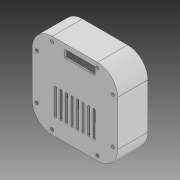
# Autodesk Inventor part: J1_Base
Saved by Autodesk Inventor 2020 (Build 240168000, 168)
## iProperties
Created: 2021-03-23
Part Number: J1_Base
Material: Generic
Document SubType Name: Modeling
Designer: DDeGo
Density: 1 g/cm^3
Appearance: Default
Author: DDeGo
Autodesk Inventor part; units mm, degrees
ref_plane "YZ Plane" through (0, 0, 0) normal (1, 0, 0) x (0, 1, 0)
ref_plane "XZ Plane" through (0, 0, 0) normal (0, 1, 0) x (-1, 0, 0)
ref_plane "XY Plane" through (0, 0, 0) normal (0, 0, 1) x (1, 0, 0)
sketch "Block1" plane through (0, 0, 0) normal (0, 0, 1) x (1, 0, 0)
  circle A0 centre (112.1187, 97.7562) radius 2.75
  line L0 (90.8687, 90.2562) -> (90.8687, 49.9679) construction
  circle A1 centre (83.3687, 50.2562) radius 2.75
  line L1 (75.8687, 49.9679) -> (75.8687, 122.7562) construction
  line L2 (75.8687, 49.9679) -> (90.8687, 49.9679) construction
  circle A2 centre (83.3687, 115.2562) radius 2.75
  line L3 (90.8687, 90.2562) -> (190.8687, 90.2562) construction
  line L4 (75.8687, 122.7562) -> (205.8687, 122.7562) construction
  circle A3 centre (140.8687, 115.2562) radius 2.75
  circle A4 centre (169.6187, 97.7562) radius 2.75
  circle A5 centre (198.3687, 115.2562) radius 2.75
  line L5 (190.8687, 90.2562) -> (190.8687, 40.2562) construction
  line L6 (205.8687, 40.2562) -> (205.8687, 122.7562) construction
  circle A6 centre (198.3687, 50.2562) radius 2.75
  line L7 (205.8687, 40.2562) -> (190.8687, 40.2562) construction
  line L8 (83.3687, 115.2562) -> (140.8687, 115.2562) construction
  line L9 (140.8687, 115.2562) -> (198.3687, 115.2562) construction
  line L10 (198.3687, 115.2562) -> (198.3687, 50.2562) construction
  line L11 (198.3687, 50.2562) -> (83.3687, 50.2562) construction
  line L12 (83.3687, 50.2562) -> (83.3687, 115.2562) construction
  line L13 (112.1187, 115.2562) -> (112.1187, 97.7562) construction
  line L14 (169.6187, 115.2562) -> (169.6187, 97.7562) construction
  line L15 (169.6187, 97.7562) -> (112.1187, 97.7562) construction
  point P0 (142.3997, 87.8737)
  point P1 (140.8687, 90.2562)
  point P2 (140.8687, 90.2562)
  dimension "d9" = 5.5
  dimension "d10" = 57.5
  dimension "d11" = 7.5
  dimension "d12" = 7.5
  dimension "d13" = 7.5
  dimension "d14" = 17.5
  dimension "d15" = 7.5
  dimension "d16" = 10
  dimension "d17" = 65
  dimension "d18" = 7.5
  dimension "d19" = 7.5
  measures "d9" diameter of A0
  measures "d10" distance of L8.start L8.end
  measures "d11" distance between parallel lines of L6 L10
  measures "d12" distance between parallel lines of L4 L9
  measures "d13" distance between parallel lines of L1 L12
  measures "d14" distance of L13.start L13.end
  measures "d15" distance between parallel lines of L3 L15
  measures "d16" distance between parallel lines of L7 L11
  measures "d17" distance of L9.end L10.end
  measures "d18" distance from line of L5 L10.end
  measures "d19" distance between parallel lines of L12 L0
sketch "Sketch1" plane through (0, 0, 0) normal (0, 0, 1) x (1, 0, 0)
  line L0 (45, -85) -> (-45, -85)
  line L1 (-85, -45) -> (-85, 45)
  line L2 (-45, 85) -> (45, 85)
  line L3 (85, 45) -> (85, -45)
  line L4 (85, -85) -> (-85, 85) construction
  line L5 (-85, -85) -> (85, 85) construction
  arc A0 (-45, 85) -> (-85, 45) centre (-45, 45) ccw
  arc A1 (85, 45) -> (45, 85) centre (45, 45) ccw
  arc A2 (45, -85) -> (85, -45) centre (45, -45) ccw
  arc A3 (-85, -45) -> (-45, -85) centre (-45, -45) ccw
  point P0 (0, 0)
  dimension "d1" = 170
  dimension "d2" = 170
  dimension "d3" = 40
  constraints: 12 end point, 8 point on circle, 8 point on line, 8 tangent, 4 centre point, 3 equal radius, 2 midpoint, 2 parallel, 1 horizontal, 1 perpendicular
  measures "d1" distance between parallel lines of L3 L1
  measures "d2" distance between parallel lines of L0 L2
  measures "d3" radius of A0
extrude "Extrusion1" add sketch "Sketch1" along normal blind 60
sketch "Sketch2" plane through (0, 0, 60) normal (0, 0, 1) x (1, 0, 0)
  line L0 (0, 0) -> (-85, 0) construction
  line L1 (-85, 45) -> (-85, -45) projected
  line L2 (0, 0) -> (0, 52.5) construction
  line L3 (45, 85) -> (-45, 85) projected
  circle A0 centre (-28.75, 60) radius 2.75
  line L4 (-50, 52.5) -> (-50, 12.2116) construction
  circle A1 centre (-57.5, 12.5) radius 2.75
  line L5 (-65, 12.2116) -> (-65, 85) construction
  line L6 (-65, 12.2116) -> (-50, 12.2116) construction
  circle A2 centre (-57.5, 77.5) radius 2.75
  line L7 (-50, 52.5) -> (50, 52.5) construction
  line L8 (-65, 85) -> (65, 85) construction
  circle A3 centre (0, 77.5) radius 2.75
  circle A4 centre (28.75, 60) radius 2.75
  circle A5 centre (57.5, 77.5) radius 2.75
  line L9 (50, 52.5) -> (50, 2.5) construction
  line L10 (65, 2.5) -> (65, 85) construction
  circle A6 centre (57.5, 12.5) radius 2.75
  line L11 (65, 2.5) -> (50, 2.5) construction
  line L12 (-57.5, 77.5) -> (0, 77.5) construction
  line L13 (0, 77.5) -> (57.5, 77.5) construction
  line L14 (57.5, 77.5) -> (57.5, 12.5) construction
  line L15 (57.5, 12.5) -> (-57.5, 12.5) construction
  line L16 (-57.5, 12.5) -> (-57.5, 77.5) construction
  line L17 (-28.75, 77.5) -> (-28.75, 60) construction
  line L18 (28.75, 77.5) -> (28.75, 60) construction
  line L19 (28.75, 60) -> (-28.75, 60) construction
  circle A7 centre (-28.75, -60) radius 2.75
  line L20 (-50, -52.5) -> (-50, -12.2116) construction
  circle A8 centre (-57.5, -12.5) radius 2.75
  line L21 (-65, -12.2116) -> (-65, -85) construction
  line L22 (-65, -12.2116) -> (-50, -12.2116) construction
  circle A9 centre (-57.5, -77.5) radius 2.75
  line L23 (-50, -52.5) -> (50, -52.5) construction
  line L24 (-65, -85) -> (65, -85) construction
  circle A10 centre (0, -77.5) radius 2.75
  circle A11 centre (28.75, -60) radius 2.75
  circle A12 centre (57.5, -77.5) radius 2.75
  line L25 (50, -52.5) -> (50, -2.5) construction
  line L26 (65, -2.5) -> (65, -85) construction
  circle A13 centre (57.5, -12.5) radius 2.75
  line L27 (65, -2.5) -> (50, -2.5) construction
  line L28 (-57.5, -77.5) -> (0, -77.5) construction
  line L29 (0, -77.5) -> (57.5, -77.5) construction
  line L30 (57.5, -77.5) -> (57.5, -12.5) construction
  line L31 (57.5, -12.5) -> (-57.5, -12.5) construction
  line L32 (-57.5, -12.5) -> (-57.5, -77.5) construction
  line L33 (-28.75, -77.5) -> (-28.75, -60) construction
  line L34 (28.75, -77.5) -> (28.75, -60) construction
  line L35 (28.75, -60) -> (-28.75, -60) construction
  constraints: 4 end point, 2 horizontal, 1 midpoint, 1 vertical, 2 other
extrude "Extrusion2" [suppressed]
ref_plane "Work Plane1" through (0, 0, -15) normal (0, 0, -1) x (-1, 0, 0)
sketch "Sketch3" plane through (0, 0, -15) normal (0, 0, -1) x (-1, 0, 0)
  circle A0 centre (0, 0) radius 87.5
  line L0 (-85, -45) -> (-85, 45) construction
  dimension "d27" = 175
  constraints: 1 centre point, 1 coincident
  measures "d27" diameter of A0
sketch "Sketch4" plane through (0, 0, 0) normal (0, 0, -1) x (-1, 0, 0)
  line L0 (-85, -45) -> (-85, 45) projected
  arc A0 (-85, -45) -> (-45, -85) centre (-45, -45) ccw projected
  line L1 (45, -85) -> (-45, -85) projected
  arc A1 (45, -85) -> (85, -45) centre (45, -45) ccw projected
  line L2 (85, 45) -> (85, -45) projected
  arc A2 (85, 45) -> (45, 85) centre (45, 45) ccw projected
  line L3 (-45, 85) -> (45, 85) projected
  arc A3 (-45, 85) -> (-85, 45) centre (-45, 45) ccw projected
  point P0 (0, 0)
loft "Loft1" add profiles "Sketch3", "Sketch4"
sketch "Sketch5" plane through (0, 0, -15) normal (0, 0, -1) x (-1, 0, 0)
  arc A0 (-37.1204, 79.2359) -> (-77.3314, 40.9402) centre (0, 0) ccw projected
  arc A1 (-77.3314, 40.9402) -> (-77.3314, -40.9402) centre (0, 0) ccw projected
  arc A2 (-77.3314, -40.9402) -> (-40.9402, -77.3314) centre (0, 0) ccw projected
  arc A3 (-40.9402, -77.3314) -> (40.9402, -77.3314) centre (0, 0) ccw projected
  arc A4 (40.9402, -77.3314) -> (77.3314, -40.9402) centre (0, 0) ccw projected
  arc A5 (77.3314, -40.9402) -> (77.3314, 40.9402) centre (0, 0) ccw projected
  arc A6 (77.3314, 40.9402) -> (40.9402, 77.3314) centre (0, 0) ccw projected
  arc A7 (40.9402, 77.3314) -> (-37.1204, 79.2359) centre (0, 0) ccw projected
extrude "Extrusion3" add sketch "Sketch5" along normal blind 5
ref_plane "Work Plane2" through (0, 0, 57) normal (0, 0, 1) x (1, 0, 0)
sketch "Sketch6" plane through (0, 0, 57) normal (0, 0, 1) x (1, 0, 0)
  arc A0 (-45, 85) -> (-85, 45) centre (-45, 45) ccw projected
  line L0 (-85, 45) -> (-85, -45) projected
  arc A1 (-85, -45) -> (-45, -85) centre (-45, -45) ccw projected
  line L1 (-45, -85) -> (45, -85) projected
  arc A2 (45, -85) -> (85, -45) centre (45, -45) ccw projected
  line L2 (85, -45) -> (85, 45) projected
  arc A3 (85, 45) -> (45, 85) centre (45, 45) ccw projected
  line L3 (45, 85) -> (-45, 85) projected
  line L4 (-81, -45) -> (-81, 45)
  arc A4 (-45, 81) -> (-81, 45) centre (-45, 45) ccw
  line L5 (-45, 81) -> (45, 81)
  arc A5 (81, 45) -> (45, 81) centre (45, 45) ccw
  line L6 (81, 45) -> (81, -45)
  arc A6 (45, -81) -> (81, -45) centre (45, -45) ccw
  line L7 (45, -81) -> (-45, -81)
  arc A7 (-81, -45) -> (-45, -81) centre (-45, -45) ccw
  line L8 (-85, 45) -> (-85, -45) projected
  point P0 (0, 0)
  dimension "d29" = 4
  constraints: 8 end point, 8 point on circle, 4 centre point, 7 other
  measures "d29" distance between parallel lines of L8 L4
ref_plane "Work Plane3" through (85, -45, 0) normal (0, 0, -1) x (-1, 0, 0)
sketch "Sketch7" plane through (85, -45, 0) normal (0, 0, -1) x (-1, 0, 0)
  arc A0 (170, 90) -> (130, 130) centre (130, 90) ccw projected
  line L0 (170, 90) -> (170, 0) projected
  arc A1 (130, -40) -> (170, 0) centre (130, 0) ccw projected
  line L1 (130, -40) -> (40, -40) projected
  arc A2 (0, 0) -> (40, -40) centre (40, 0) ccw projected
  line L2 (0, 0) -> (0, 90) projected
  arc A3 (40, 130) -> (0, 90) centre (40, 90) ccw projected
  line L3 (40, 130) -> (130, 130) projected
  line L4 (166, 0) -> (166, 90)
  arc A4 (166, 90) -> (130, 126) centre (130, 90) ccw
  line L5 (130, 126) -> (40, 126)
  arc A5 (40, 126) -> (4, 90) centre (40, 90) ccw
  line L6 (4, 90) -> (4, 0)
  arc A6 (4, 0) -> (40, -36) centre (40, 0) ccw
  line L7 (40, -36) -> (130, -36)
  arc A7 (130, -36) -> (166, 0) centre (130, 0) ccw
  point P0 (85, 45)
  dimension "d30" = 4
  constraints: 8 end point, 8 point on circle, 4 centre point, 7 other
  measures "d30" distance between parallel lines of L0 L4
extrude "Extrusion4" cut sketch "Sketch6" against normal up to surface (57 mm away) contours L4 A4 L5 A5 L6 A6 L7 A7
sketch "Sketch8" plane through (0, 0, -20) normal (0, 0, -1) x (-1, 0, 0)
  circle A0 centre (0, 0) radius 72.5
  dimension "d33" = 145
  constraints: 1 centre point, 1 coincident
  measures "d33" diameter of A0
extrude "Extrusion5" cut sketch "Sketch8" against normal blind 29.75
sketch "Sketch9" plane through (-81, -45, 57) normal (-1, 0, 0) x (0, 0, 1)
  line L0 (-13.6892, 69.9987) -> (-53.6892, 69.9987) construction
  line L1 (-53.6892, 69.9987) -> (-53.6892, 29.9987) construction
  line L2 (-53.6892, 29.9987) -> (-13.6892, 29.9987) construction
  line L3 (-13.6892, 29.9987) -> (-13.6892, 69.9987) construction
  line L4 (-13.6892, 69.9987) -> (-53.6892, 29.9987) construction
  line L5 (-53.6892, 69.9987) -> (-13.6892, 29.9987) construction
  circle A0 centre (-33.6892, 49.9987) radius 19
  point P0 (-57, 45)
  dimension "d36" = 40
  dimension "d37" = 40
  dimension "d38" = 38
  constraints: 12 end point, 2 midpoint, 2 parallel, 1 centre point, 1 coincident, 1 horizontal, 1 perpendicular
  measures "d36" distance of L0.end L1.end
  measures "d37" distance of L1.end L2.end
  measures "d38" diameter of A0
extrude "Extrusion6" cut sketch "Sketch9" along normal through all
sketch "Sketch10" plane through (0, 0, 57) normal (0, 0, -1) x (-1, 0, 0)
  line L0 (20, 60.5) -> (-40, 60.5)
  line L1 (-40, 60.5) -> (-40, 75.4)
  line L2 (-40, 75.4) -> (20, 75.4)
  line L3 (20, 75.4) -> (20, 60.5)
  line L4 (-45, 85) -> (45, 85) projected
  point P0 (0, 0)
  point P1 (0, 85)
  dimension "d69" = 9.6
  dimension "d70" = 24.5
  dimension "d71" = 20
  dimension "d72" = 40
  constraints: 8 end point, 2 parallel, 1 horizontal, 1 midpoint, 1 perpendicular
  measures "d69" distance between parallel lines of L4 L2
  measures "d70" distance between parallel lines of L4 L0
  measures "d71" distance from line of L3 point (0, 85)
  measures "d72" distance from line of L1 point (0, 85)
extrude "Extrusion7" cut sketch "Sketch10" against normal through all
sketch "Sketch11" plane through (0, 0, 60) normal (0, 0, 1) x (1, 0, 0)
  line L0 (-38.2933, -49.6427) -> (-38.2933, 0.3573) construction
  line L1 (-40.2933, -49.6427) -> (-40.2933, 0.3573)
  line L2 (-36.2933, 0.3573) -> (-36.2933, -49.6427)
  arc A0 (-40.2933, -49.6427) -> (-36.2933, -49.6427) centre (-38.2933, -49.6427) ccw
  arc A1 (-36.2933, 0.3573) -> (-40.2933, 0.3573) centre (-38.2933, 0.3573) ccw
  line L3 (0, 0) -> (68.8945, 0) construction
  line L4 (-27.2933, -49.6427) -> (-27.2933, 0.3573) construction
  line L5 (-29.2933, -49.6427) -> (-29.2933, 0.3573)
  line L6 (-25.2933, 0.3573) -> (-25.2933, -49.6427)
  arc A2 (-29.2933, -49.6427) -> (-25.2933, -49.6427) centre (-27.2933, -49.6427) ccw
  arc A3 (-25.2933, 0.3573) -> (-29.2933, 0.3573) centre (-27.2933, 0.3573) ccw
  line L7 (-16.2933, -49.6427) -> (-16.2933, 0.3573) construction
  line L8 (-18.2933, -49.6427) -> (-18.2933, 0.3573)
  line L9 (-14.2933, 0.3573) -> (-14.2933, -49.6427)
  arc A4 (-18.2933, -49.6427) -> (-14.2933, -49.6427) centre (-16.2933, -49.6427) ccw
  arc A5 (-14.2933, 0.3573) -> (-18.2933, 0.3573) centre (-16.2933, 0.3573) ccw
  line L10 (-5.2933, -49.6427) -> (-5.2933, 0.3573) construction
  line L11 (-7.2933, -49.6427) -> (-7.2933, 0.3573)
  line L12 (-3.2933, 0.3573) -> (-3.2933, -49.6427)
  arc A6 (-7.2933, -49.6427) -> (-3.2933, -49.6427) centre (-5.2933, -49.6427) ccw
  arc A7 (-3.2933, 0.3573) -> (-7.2933, 0.3573) centre (-5.2933, 0.3573) ccw
  line L13 (5.7067, -49.6427) -> (5.7067, 0.3573) construction
  line L14 (3.7067, -49.6427) -> (3.7067, 0.3573)
  line L15 (7.7067, 0.3573) -> (7.7067, -49.6427)
  arc A8 (3.7067, -49.6427) -> (7.7067, -49.6427) centre (5.7067, -49.6427) ccw
  arc A9 (7.7067, 0.3573) -> (3.7067, 0.3573) centre (5.7067, 0.3573) ccw
  line L16 (16.7067, -49.6427) -> (16.7067, 0.3573) construction
  line L17 (14.7067, -49.6427) -> (14.7067, 0.3573)
  line L18 (18.7067, 0.3573) -> (18.7067, -49.6427)
  arc A10 (14.7067, -49.6427) -> (18.7067, -49.6427) centre (16.7067, -49.6427) ccw
  arc A11 (18.7067, 0.3573) -> (14.7067, 0.3573) centre (16.7067, 0.3573) ccw
  line L19 (27.7067, -49.6427) -> (27.7067, 0.3573) construction
  line L20 (25.7067, -49.6427) -> (25.7067, 0.3573)
  line L21 (29.7067, 0.3573) -> (29.7067, -49.6427)
  arc A12 (25.7067, -49.6427) -> (29.7067, -49.6427) centre (27.7067, -49.6427) ccw
  arc A13 (29.7067, 0.3573) -> (25.7067, 0.3573) centre (27.7067, 0.3573) ccw
  line L22 (38.7067, -49.6427) -> (38.7067, 0.3573) construction
  line L23 (36.7067, -49.6427) -> (36.7067, 0.3573)
  line L24 (40.7067, 0.3573) -> (40.7067, -49.6427)
  arc A14 (36.7067, -49.6427) -> (40.7067, -49.6427) centre (38.7067, -49.6427) ccw
  arc A15 (40.7067, 0.3573) -> (36.7067, 0.3573) centre (38.7067, 0.3573) ccw
  point P0 (-38.2933, -24.6427)
  point P1 (-27.2933, -24.6427)
  point P2 (-16.2933, -24.6427)
  point P3 (-5.2933, -24.6427)
  point P4 (5.7067, -24.6427)
  point P5 (16.7067, -24.6427)
  point P6 (27.7067, -24.6427)
  point P7 (38.7067, -24.6427)
  dimension "d43" = 50
  dimension "d44" = 2
  dimension "d47" = 11
  constraints: 66 end point, 32 point on circle, 16 centre point, 4 tangent, 2 horizontal, 1 midpoint, 1 parallel, 1 vertical, 84 other
  measures "d43" distance of L0.start L0.end
  measures "d44" radius of A1
  measures "d47" distance of L1.start L5.start
extrude "Extrusion8" cut sketch "Sketch11" against normal blind 10
sketch "Sketch12" plane through (-45, 81, 0) normal (0, 0, 1) x (1, 0, 0)
  circle A0 centre (38.7385, -72.8833) radius 193.3593
  point P0 (45, -81)
  constraints: 1 centre point
extrude "SnipSnip" cut sketch "Sketch12" against normal through all
sketch "Sketch13" plane through (-45, -85, 60) normal (0, -1, 0) x (1, 0, 0)
  line L0 (-0.9101, -8.6737) -> (19.7466, -8.6737)
  line L1 (19.7466, -8.6737) -> (19.7466, -23.4777)
  line L2 (19.7466, -23.4777) -> (-0.9101, -23.4777)
  line L3 (-0.9101, -23.4777) -> (-0.9101, -8.6737)
  line L4 (61.8635, -8.6737) -> (77.0118, -8.6737)
  line L5 (77.0118, -8.6737) -> (77.0118, -15.7888)
  line L6 (77.0118, -15.7888) -> (61.8635, -15.7888)
  line L7 (61.8635, -15.7888) -> (61.8635, -8.6737)
  point P0 (45, -60)
  constraints: 16 end point, 4 parallel, 2 horizontal, 2 perpendicular, 1 point on line
extrude "Extrusion10" cut sketch "Sketch13" against normal blind 10
sketch "Sketch14" plane through (-45, 81, 0) normal (0, 0, -1) x (-1, 0, 0)
  arc A0 (0, -162) -> (36, -126) centre (0, -126) ccw projected
  line L0 (0, -162) -> (-90, -162) projected
  arc A1 (-126, -126) -> (-90, -162) centre (-90, -126) ccw projected
  line L1 (-126, -126) -> (-126, -36) projected
  arc A2 (-90, 0) -> (-126, -36) centre (-90, -36) ccw projected
  line L2 (-90, 0) -> (0, 0) projected
  arc A3 (36, -36) -> (0, 0) centre (0, -36) ccw projected
  line L3 (36, -36) -> (36, -126) projected
  arc A4 (-90, 4) -> (-130, -36) centre (-90, -36) ccw projected
  line L4 (-130, -126) -> (-130, -36) projected
  arc A5 (-130, -126) -> (-90, -166) centre (-90, -126) ccw projected
  line L5 (0, -166) -> (-90, -166) projected
  arc A6 (0, -166) -> (40, -126) centre (0, -126) ccw projected
  line L6 (40, -36) -> (40, -126) projected
  arc A7 (40, -36) -> (0, 4) centre (0, -36) ccw projected
  line L7 (-90, 4) -> (0, 4) projected
  line L8 (-90, -36) -> (-90, -5.5) construction
  line L9 (-90, -36) -> (-120.5, -36) construction
  line L10 (-90, -36) -> (-45, -81) construction
  circle A8 centre (-120.5, -36) radius 3.1
  circle A9 centre (-90, -5.5) radius 3.1
  arc A10 (-95.5, -5.5) -> (-84.5, -5.5) centre (-90, -5.5) ccw
  line L11 (-90, 0) -> (0, 0) projected
  arc A11 (-120.5, -41.5) -> (-120.5, -30.5) centre (-120.5, -36) ccw
  line L12 (-126, -126) -> (-126, -36) projected
  line L13 (-120.5, -41.5) -> (-126, -41.5)
  line L14 (-120.5, -30.5) -> (-126, -30.5)
  line L15 (-95.5, -5.5) -> (-95.5, 0)
  line L16 (-84.5, -5.5) -> (-84.5, 0)
  line L17 (-84.5, -156.5) -> (-84.5, -162)
  arc A12 (-84.5, -156.5) -> (-95.5, -156.5) centre (-90, -156.5) ccw
  line L18 (-95.5, -156.5) -> (-95.5, -162)
  circle A13 centre (-90, -156.5) radius 3.1
  line L19 (-120.5, -120.5) -> (-126, -120.5)
  arc A14 (-120.5, -131.5) -> (-120.5, -120.5) centre (-120.5, -126) ccw
  circle A15 centre (-120.5, -126) radius 3.1
  line L20 (-120.5, -131.5) -> (-126, -131.5)
  line L21 (30.5, -120.5) -> (36, -120.5)
  arc A16 (30.5, -120.5) -> (30.5, -131.5) centre (30.5, -126) ccw
  line L22 (30.5, -131.5) -> (36, -131.5)
  circle A17 centre (30.5, -126) radius 3.1
  line L23 (-5.5, -156.5) -> (-5.5, -162)
  arc A18 (5.5, -156.5) -> (-5.5, -156.5) centre (0, -156.5) ccw
  circle A19 centre (0, -156.5) radius 3.1
  line L24 (5.5, -156.5) -> (5.5, -162)
  line L25 (-5.5, -5.5) -> (-5.5, 0)
  arc A20 (-5.5, -5.5) -> (5.5, -5.5) centre (0, -5.5) ccw
  line L26 (5.5, -5.5) -> (5.5, 0)
  circle A21 centre (0, -5.5) radius 3.1
  line L27 (30.5, -41.5) -> (36, -41.5)
  arc A22 (30.5, -30.5) -> (30.5, -41.5) centre (30.5, -36) ccw
  circle A23 centre (30.5, -36) radius 3.1
  line L28 (30.5, -30.5) -> (36, -30.5)
  point P0 (-90, -162)
  point P1 (-90, -166)
  point P2 (-126, -126)
  point P3 (-130, -126)
  point P4 (36, -126)
  point P5 (40, -126)
  point P6 (0, -166)
  point P7 (0, 0)
  point P8 (0, 4)
  point P9 (36, -36)
  point P10 (40, -36)
  point P11 (36, -41.5)
  point P12 (35.5774, -30.5)
  point P13 (35.5774, -131.5)
  point P14 (36, -120.5)
  point P15 (-125.5774, -131.5)
  point P16 (-125.5774, -30.5)
  point P17 (-126, -41.5)
  point P18 (-84.5, 0)
  point P19 (-95.5, -0.4226)
  point P20 (5.5, -0.4226)
  point P21 (-5.5, 0)
  point P22 (-5.5, -162)
  point P23 (5.5, -161.5774)
  point P24 (-95.5, -161.5774)
  point P25 (-84.5, -162)
  dimension "d58" = 5.5
  dimension "d59" = 45
  dimension "d60" = 6.2
  dimension "d63" = 360
  dimension "d73" = 9.5
  constraints: 38 end point, 16 centre point, 16 coincident, 16 point on circle, 6 tangent, 5 perpendicular, 4 point on line, 1 equal radius, 106 other
  measures "d58" distance from line of L2 L8.end
  measures "d59" angle of L10 L8
  measures "d60" diameter of A9
  measures "d73" distance from line of L7 L8.end
extrude "Extrusion11" add sketch "Sketch14" against normal up to surface (57 mm away) contours L0 L23 A18 L24 A0 | L22 A16 L21 L3 A0 | L0 A1 L18 A12 L17 | L27 A22 L28 A3 L3 | A1 L1 L19 A14 L20 | L26 A20 L25 L2 A3 | L1 A2 L14 A11 L13 | L16 A10 L15 A2 L2
sketch "Sketch15" plane through (-45, 81, 0) normal (0, 0, -1) x (-1, 0, 0)
  circle A0 centre (-120.5, -36) radius 3.1 projected
  circle A1 centre (-120.5, -126) radius 3.1 projected
  circle A2 centre (30.5, -126) radius 3.1 projected
  circle A3 centre (30.5, -36) radius 3.1 projected
  circle A4 centre (-90, -156.5) radius 3.1 projected
  circle A5 centre (0, -156.5) radius 3.1 projected
  circle A6 centre (-90, -5.5) radius 3.1 projected
  circle A7 centre (0, -5.5) radius 3.1 projected
  point P0 (-45, -81)
extrude "Extrusion12" cut sketch "Sketch15" against normal through all
equation "\"d12\" = d11"
equation "\"d13\" = d11"
equation "\"d15\" = d11"
equation "\"d18\" = d11"
equation "\"d19\" = d11"
body "Solid1"
